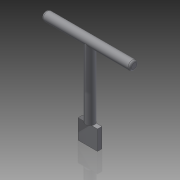
# Autodesk Inventor part: Flutschlüssel
Saved by Autodesk Inventor 2015 SP2 (Build 190223200, 223)
## iProperties
Created: 2016-11-08
Part Number: Flutschlüssel
Material: Allgemein
Document SubType Name: Modeling
Designer: Gruber
Density: 1 g/cm^3
Appearance: Vorgabe
Project: Neuer Ordner
RuleStatus: InUse
AfterDocSave0: file://Projektnummer
And.-Index: 0
Dateiname: Flutschlüssel
Author: Gruber
Autodesk Inventor part; units mm, degrees
ref_plane "XZ Plane" through (0, 0, 0) normal (0, 1, 0) x (-1, 0, 0)
ref_plane "XY Plane" through (0, 0, 0) normal (0, 0, 1) x (1, 0, 0)
sketch "Skizze1" plane through (0, 0, 0) normal (0, 0, 1) x (1, 0, 0)
  line L0 (-14, -11) -> (14, -11)
  line L1 (14, -11) -> (14, 11)
  line L2 (14, 11) -> (-14, 11)
  line L3 (-14, 11) -> (-14, -11)
  line L4 (-14, -11) -> (14, 11) construction
  line L5 (14, -11) -> (-14, 11) construction
  point P0 (0, 0)
  dimension "d0" = 28
  dimension "d1" = 22
  constraints: 12 end point, 2 midpoint, 2 parallel, 1 horizontal, 1 perpendicular
  measures "d0" distance of L2.end L1.end
  measures "d1" distance of L1.end L0.end
extrude "Extrusion1" add sketch "Skizze1" along normal blind 6
sketch "Skizze2" plane through (-14, 11, 0) normal (0, 1, 0) x (1, 0, 0)
  circle A0 centre (14, -3) radius 5
  line L0 (0, 0) -> (0, -6) projected
  line L1 (28, 0) -> (0, 0) projected
  point P0 (14, 0)
  point P1 (0, -3)
  point P2 (14, 0)
  dimension "d4" = 10
  constraints: 2 midpoint, 1 centre point, 1 horizontal alignment, 1 vertical alignment
  measures "d4" diameter of A0
extrude "Extrusion2" add sketch "Skizze2" along normal blind 80
ref_plane "Arbeitsebene1" through (0, 0, 0) normal (1, 0, 0) x (0, 1, 0)
sketch "Skizze3" plane through (0, 0, 0) normal (1, 0, 0) x (0, 1, 0)
  line L0 (91, -2) -> (91, 8) projected
  circle A0 centre (91, 3) radius 5
  point P0 (0, 0)
  dimension "d8" = 10
  constraints: 1 centre point, 1 midpoint
  measures "d8" diameter of A0
extrude "Extrusion3" add sketch "Skizze3" along normal mid plane 100
fillet "Rundung1" radius 2 2 edges at (50, 86, 3) (-50, 86, 3)
